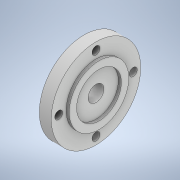
# Autodesk Inventor part: Part4
Saved by Autodesk Inventor 2021 (Build 250183000, 183)
## iProperties
Created: 2022-06-05
Part Number: Part4
Material: Generic
Document SubType Name: Modeling
Designer: Bhargav Malasani
Density: 1 g/cm^3
Appearance: Default
Author: Bhargav Malasani
Autodesk Inventor part; units mm, degrees
ref_plane "YZ Plane" through (0, 0, 0) normal (1, 0, 0) x (0, 1, 0)
ref_plane "XZ Plane" through (0, 0, 0) normal (0, 1, 0) x (-1, 0, 0)
ref_plane "XY Plane" through (0, 0, 0) normal (0, 0, 1) x (1, 0, 0)
sketch "Sketch1" plane through (0, 0, 0) normal (1, 0, 0) x (0, 1, 0)
  circle A0 centre (0, 0) radius 45
  dimension "d0" = 90
  constraints: 1 centre point, 1 coincident
  measures "d0" diameter of A0
extrude "Extrusion1" add sketch "Sketch1" along normal mid plane 12
sketch "Sketch2" plane through (6, 0, 0) normal (1, 0, 0) x (0, 0, -1)
  circle A0 centre (0, 0) radius 30
  circle A1 centre (0, 0) radius 22.5
  dimension "d3" = 60
  dimension "d4" = 45
  constraints: 2 centre point, 2 coincident
  measures "d3" diameter of A0
  measures "d4" diameter of A1
extrude "Extrusion2" add sketch "Sketch2" along normal blind 3
sketch "Sketch3" plane through (-6, 0, 0) normal (-1, 0, 0) x (0, 0, 1)
  circle A0 centre (0, 0) radius 19
  dimension "d7" = 38
  constraints: 1 centre point, 1 coincident
  measures "d7" diameter of A0
extrude "Extrusion3" add sketch "Sketch3" along normal blind 3
sketch "Sketch4" plane through (6, 0, 0) normal (1, 0, 0) x (0, 0, -1)
  circle A0 centre (0, 0) radius 8
  circle A1 centre (0, 37.5) radius 4
  circle A2 centre (-37.5, 0) radius 4
  circle A3 centre (0, -37.5) radius 4
  circle A4 centre (37.5, 0) radius 4
  dimension "d10" = 16
  dimension "d11" = 8
  dimension "d12" = 37.5
  dimension "d15" = 360
  dimension "d17" = 75
  dimension "d18" = 37.5
  constraints: 5 centre point, 1 coincident, 9 other
  measures "d10" diameter of A0
  measures "d11" diameter of A1
  measures "d12" distance of point (0, 0) A1.centre
  measures "d17" distance of A3.centre A1.centre
  measures "d18" distance of A2.centre point (0, 0)
extrude "Extrusion4" cut sketch "Sketch4" against normal through all
body "Solid1"
